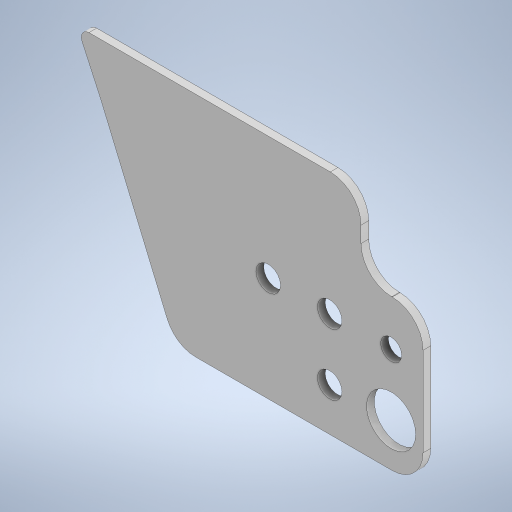
# Autodesk Inventor part: Sleds poly V3
Saved by Autodesk Inventor 2023 (Build 270158000, 158)
## iProperties
Created: 2024-01-28
Part Number: Sleds poly V3
Material: Generic
Document SubType Name: Modeling
Designer: diego
Density: 1 g/cm^3
Appearance: Default
Author: diego
Autodesk Inventor part; units mm, degrees
ref_plane "YZ Plane" through (0, 0, 0) normal (1, 0, 0) x (0, 1, 0)
ref_plane "XZ Plane" through (0, 0, 0) normal (0, 1, 0) x (-1, 0, 0)
ref_plane "XY Plane" through (0, 0, 0) normal (0, 0, 1) x (1, 0, 0)
sketch "Sketch2" plane through (0, 0, 0) normal (0, 0, 1) x (1, 0, 0)
  line L0 (39.8575, 12.7612) -> (31.599, 12.7612)
  line L1 (39.8575, 12.7612) -> (20.8075, 12.7612)
  line L2 (79.512, -31.9773) -> (79.512, 12.7612)
  line L3 (79.512, 12.7612) -> (37.4294, 12.7612)
  circle A0 centre (60.3451, -12.7) radius 2.54
  circle A1 centre (73.0451, -12.7) radius 2.54
  circle A2 centre (73.0451, -25.4) radius 2.54
  line L4 (92.334, -18.8499) -> (92.334, 1.5256)
  circle A3 centre (85.7451, -25.4) radius 3.9624
  circle A4 centre (85.7451, -12.7) radius 2.1844
  line L5 (25.7365, 2.0147) -> (43.2474, -39.355)
  line L6 (47.6451, -34.29) -> (41.1035, -34.29)
  line L7 (92.334, -18.8499) -> (92.334, -34.29)
  line L8 (47.6451, -34.29) -> (92.334, -34.29)
  line L9 (-341.1851, -3.2325) -> (91.1147, -3.2325)
  line L10 (25.7365, 2.0147) -> (20.8075, 12.7612)
  line L11 (91.1147, -3.2325) -> (92.334, -3.2325)
  circle A5 centre (85.7451, -25.4) radius 5.08
  point P0 (0, 0)
  point P1 (41.3274, -31.9773)
  point P2 (79.512, -18.8499)
  point P3 (79.512, -3.2325)
  dimension "d38" = 19.05
  dimension "d39" = 432.2999
  dimension "d40" = 10.16
  constraints: 24 end point, 6 centre point, 6 point on line, 4 horizontal, 1 coincident, 1 perpendicular, 1 vertical
  measures "d38" distance of L0.start L1.end
  measures "d39" distance of L9.start L9.end
  measures "d40" diameter of A5
extrude "Extrusion3" add sketch "Sketch2" along normal blind 1.5875 contours L3 L2 L9 L5 L10 L1 L0 | L9 L11 L4 L7 L8 L6 L5
fillet "Fillet9" radius 6.35 5 edges at (79.512, 12.7612, 0.7937) (79.512, -3.2325, 0.7937) (92.334, -3.2325, 0.7937) (92.334, -34.29, 0.7937) (41.1035, -34.29, 0.7937)
fillet "Fillet10" radius 1.5875 1 edges at (20.8075, 12.7612, 0.7937)
body "Solid2"
